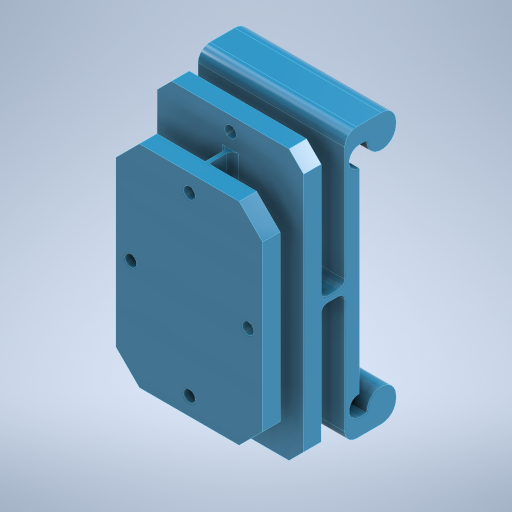
# Autodesk Inventor part: Rail-FlextureBaseLarge
Saved by Autodesk Inventor 2023.1 (Build 271208000, 208)
## iProperties
Created: 2023-06-05
Part Number: Rail-FlextureBaseLarge
Material: ABS Plastic
Document SubType Name: Modeling
Designer: hello
Density: 1.06 g/cm^3
Appearance: Sky Blue Dark
Mass: 24.8987 g
Surface Area: 148.331 cm^2
Volume: 23.4894 cm^3
Author: hello
Autodesk Inventor part; units mm, degrees
ref_plane "YZ Plane" through (0, 0, 0) normal (1, 0, 0) x (0, 1, 0)
ref_plane "XZ Plane" through (0, 0, 0) normal (0, 1, 0) x (-1, 0, 0)
ref_plane "XY Plane" through (0, 0, 0) normal (0, 0, 1) x (1, 0, 0)
sketch "Sketch1" plane through (0, 0, 0) normal (1, 0, 0) x (0, 1, 0)
  line L0 (-46, -7.5) -> (-46, 1)
  line L1 (-42, 5) -> (42, 5)
  line L2 (46, 1) -> (46, -7.5)
  line L3 (-41, -12.5) -> (-39.95, -12.5)
  line L4 (-40.25, -2.509) -> (-40.25, 0)
  line L5 (-40.25, 0) -> (40.25, 0)
  line L6 (-1, 5) -> (-1, 13)
  line L7 (-1, 13) -> (1, 13)
  line L8 (1, 13) -> (1, 5)
  line L9 (-46, 19) -> (46, 19)
  line L10 (46, 19) -> (46, 13)
  line L11 (46, 13) -> (-46, 13)
  line L12 (-46, 13) -> (-46, 19)
  arc A0 (46, 1) -> (42, 5) centre (42, 1) ccw
  arc A1 (-42, 5) -> (-46, 1) centre (-42, 1) ccw
  arc A2 (40.25, 0) -> (33.25, 0) centre (36.75, 0) ccw
  arc A3 (-33.25, 0) -> (-40.25, 0) centre (-36.75, 0) ccw
  line L13 (40.25, 0) -> (40.25, -2.509)
  arc A4 (-39.95, -12.5) -> (-40.25, -2.509) centre (-39.95, -7.5) ccw
  arc A5 (-46, -7.5) -> (-41, -12.5) centre (-41, -7.5) ccw
  circle A6 centre (39.95, -7.5) radius 5
  line L14 (41, -12.5) -> (39.95, -12.5)
  arc A7 (41, -12.5) -> (46, -7.5) centre (41, -7.5) ccw
  point P0 (0, 0)
  point P1 (-46, -12.5)
  point P2 (-46, 5)
  point P3 (46, 5)
  point P4 (46, -12.5)
  point P5 (0, 5)
  point P6 (0, 0)
  point P7 (0, 13)
  point P8 (1, 13)
  point P9 (-1, 13)
  point P10 (-40.25, -1.2545)
  point P11 (40.25, -1.2545)
  point P12 (40.25, -2.509)
  dimension "d71" = 10
  dimension "d2" = 80.5
  dimension "d10" = 92
  dimension "d11" = 5
  dimension "d13" = 2
  dimension "d14" = 8
  dimension "d15" = 6
  dimension "d52" = 4
  dimension "d53" = 7
  dimension "d54" = 7
  dimension "d67" = 10
  dimension "d68" = 7.5
  dimension "d69" = 0.3
  dimension "d70" = 5
  dimension "d72" = 0.3
  dimension "d73" = 5
  constraints: 30 end point, 14 point on circle, 14 point on line, 8 tangent, 7 centre point, 6 midpoint, 6 perpendicular, 6 vertical alignment, 3 horizontal, 3 vertical, 2 horizontal alignment, 2 parallel, 1 coincident, 1 equal radius, 3 other
  measures "d2" distance of L4.end L5.end
  measures "d10" distance of point (-46, 5) point (46, 5)
  measures "d11" distance between parallel lines of L1 L5
  measures "d13" distance of L6.end L7.end
  measures "d14" distance of L6.start L6.end
  measures "d15" distance of L11.end L9.start
  measures "d52" radius of A0
  measures "d53" distance of A2.end L5.end
  measures "d54" distance of L4.end A3.start
  measures "d67" diameter of A4
  measures "d68" distance from line of L5 A4.centre
  measures "d69" distance from line of A4.centre L4
  measures "d70" radius of A5
  measures "d72" horizontal distance of point (39.95, -7.5) point (40.25, -1.255)
  measures "d73" radius of A7
extrude "Extrusion1" add sketch "Sketch1" along normal mid plane 50 contours L0 A1 L1 A0 L2 A7 L14 A6 L13 A2 L5 A3 L4 A4 L3 A5 | L6 L7 L8 L1 | L11 L12 L9 L10 L7 | A6
sketch "Sketch2" plane through (-25, -46, 19) normal (0, 0, 1) x (1, 0, 0)
  line L0 (0, 0) -> (50, 0) projected
  line L1 (50, 92) -> (50, 0) projected
  line L2 (0, 92) -> (50, 92) projected
  line L3 (0, 0) -> (0, 92) projected
  line L4 (25.625, 10) -> (24.375, 10)
  line L5 (24.375, 10) -> (24.375, 82)
  line L6 (24.375, 82) -> (25.625, 82)
  line L7 (25.625, 82) -> (25.625, 10)
  line L8 (25.625, 10) -> (24.375, 82) construction
  line L9 (24.375, 10) -> (25.625, 82) construction
  point P0 (25, 46)
  point P1 (20.75, 0)
  point P2 (20.75, 50)
  point P3 (19.25, 50)
  point P4 (19.25, 0)
  point P5 (25, 10)
  dimension "d16" = 1.25
  dimension "d19" = 10
  constraints: 12 end point, 3 midpoint, 2 parallel, 1 horizontal, 1 perpendicular
  measures "d16" distance of L4.start L4.end
  measures "d19" distance from line of L0 point (25, 10)
extrude "Extrusion2" add sketch "Sketch2" along normal blind 8 contours L4 L5 L6 L7
sketch "Sketch3" plane through (-25, -46, 19) normal (0, 0, 1) x (1, 0, 0)
  line L0 (25.625, 82) -> (25.625, 10) projected
  line L1 (25.625, 10) -> (24.375, 10) projected
  line L2 (24.375, 10) -> (24.375, 82) projected
  line L3 (24.375, 82) -> (25.625, 82) projected
  line L4 (0, 0) -> (50, 0) projected
  line L5 (50, 92) -> (50, 0) projected
  line L6 (0, 92) -> (50, 92) projected
  line L7 (0, 0) -> (0, 92) projected
  line L8 (25.625, 10) -> (24.375, 10) projected
  line L9 (25, 10) -> (25, 0)
  line L10 (24.375, 82) -> (25.625, 82) projected
  line L11 (25, 82) -> (25, 92)
  point P0 (25, 46)
  point P1 (25, 5)
  point P2 (25, 87)
  constraints: 6 midpoint, 4 end point
hole "Hole1" at (0, -41, 19) at (0, 41, 19) direction (0, 0, -1) diameter 4 depth 8 tip angle 118
sketch "Sketch4" plane through (-25, -46, 27) normal (0, 0, 1) x (1, 0, 0)
  line L0 (0, 10) -> (50, 10)
  line L1 (50, 10) -> (50, 82)
  line L2 (50, 82) -> (0, 82)
  line L3 (0, 82) -> (0, 10)
  line L4 (0, 10) -> (50, 82) construction
  line L5 (50, 10) -> (0, 82) construction
  line L6 (25.625, 82) -> (24.375, 82) projected
  line L7 (0, 0) -> (0, 92) projected
  point P0 (25, 46)
  point P1 (25, 82)
  point P2 (0, 46)
  constraints: 12 end point, 6 midpoint, 2 parallel, 1 horizontal, 1 perpendicular
extrude "Extrusion3" add sketch "Sketch4" along normal blind 6
sketch "Sketch5" plane through (-25, -46, 33) normal (0, 0, 1) x (1, 0, 0)
  line L0 (50, 82) -> (0, 82) projected
  line L1 (0, 82) -> (0, 10) projected
  line L2 (0, 10) -> (50, 10) projected
  line L3 (50, 10) -> (50, 82) projected
  line L4 (5, 46) -> (45, 46)
  point P0 (25, 46)
  point P1 (25, 46)
  dimension "d29" = 5
  constraints: 3 coincident, 2 end point, 1 horizontal, 1 midpoint
  measures "d29" distance from line of L1 L4.start
hole "Hole2" at (-20, 0, 33) at (20, 0, 33) direction (0, 0, -1) diameter 4 depth 8 tip angle 118
sketch "Sketch6" plane through (-25, -46, 33) normal (0, 0, 1) x (1, 0, 0)
  circle A0 centre (5, 46) radius 2 projected
  circle A1 centre (45, 46) radius 2 projected
  line L0 (50, 82) -> (0, 82) projected
  line L1 (0, 82) -> (0, 10) projected
  line L2 (0, 10) -> (50, 10) projected
  line L3 (50, 10) -> (50, 82) projected
  line L4 (25, 16) -> (25, 76)
  point P0 (25, 46)
  point P1 (25, 46)
  point P2 (25, 46)
  dimension "d38" = 60
  constraints: 4 coincident, 2 end point, 1 midpoint, 1 vertical
  measures "d38" distance of L4.start L4.end
hole "Hole3" at (0, -30, 33) at (0, 30, 33) direction (0, 0, -1) diameter 4 depth 5
chamfer "Chamfer1" distance 5 angle 45 4 edges at (-25, -46, 16) (-25, 46, 16) (25, -46, 16) (25, 46, 16)
chamfer "Chamfer2" distance 8 angle 45 4 edges at (25, 36, 30) (25, -36, 30) (-25, -36, 30) (-25, 36, 30)
fillet "Fillet1" radius 2 6 edges at (0.625, 0, 19) (-0.625, 0, 19) (0, -1, 5) (0, 1, 5) (0, -1, 13) (0, 1, 13)
equation "\"d72\" = d69"
body "Solid1"
